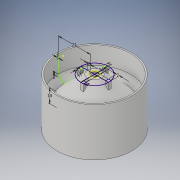
# Autodesk Inventor part: flyflipfunnel
Saved by Autodesk Inventor 2019 (Build 230136000, 136)
## iProperties
Created: 2019-02-13
Part Number: flyflipfunnel
Material: Generic
Document SubType Name: Modeling
Designer: rhaase
Density: 1 g/cm^3
Appearance: Default
Author: rhaase
Autodesk Inventor part; units mm, degrees
ref_plane "YZ Plane" through (0, 0, 0) normal (1, 0, 0) x (0, 1, 0)
ref_plane "XZ Plane" through (0, 0, 0) normal (0, 1, 0) x (-1, 0, 0)
ref_plane "XY Plane" through (0, 0, 0) normal (0, 0, 1) x (1, 0, 0)
sketch "Sketch1" plane through (0, 0, 0) normal (0, 0, 1) x (1, 0, 0)
  line L0 (-3.313, 2.109) -> (-3.313, 22.109)
  line L1 (-3.313, 4.109) -> (-3.313, 2.109)
  line L2 (22.687, -0.5116) -> (12.687, 9.4884)
  line L3 (12.687, 9.4884) -> (12.687, 7.4884)
  line L4 (12.687, 7.4884) -> (22.687, -2.5116)
  line L5 (22.687, -2.5116) -> (22.687, -0.5116)
  line L6 (-0.313, 2.109) -> (19.687, 22.109)
  line L7 (19.687, 22.109) -> (17.687, 22.109)
  line L8 (17.687, 22.109) -> (-0.313, 4.109)
  line L9 (12.187, 14.609) -> (13.6012, 16.0232)
  line L10 (-0.313, 2.109) -> (19.687, 22.109)
  line L11 (17.687, 22.109) -> (-0.313, 4.109)
  line L12 (-0.313, 4.109) -> (-0.313, 2.109)
  line L13 (19.687, 22.109) -> (17.687, 22.109)
  line L14 (-0.313, 4.109) -> (-0.313, 2.109)
  line L15 (-0.313, 2.109) -> (19.687, 22.109)
  line L16 (17.687, 22.109) -> (-0.313, 4.109)
  line L17 (-0.313, 4.109) -> (-3.313, 7.109)
  line L18 (-3.313, 22.109) -> (-4.313, 22.109)
  line L19 (-3.313, 7.109) -> (-3.313, 9.109)
  line L20 (-3.313, 9.109) -> (0.687, 5.109)
  line L21 (-3.313, 7.109) -> (-3.313, -2.5116)
  line L22 (-4.313, -2.5116) -> (-4.313, 22.109)
  line L23 (-3.313, 22.109) -> (-3.313, 9.109)
  line L24 (-4.313, -2.5116) -> (-3.313, -2.5116)
  line L25 (-4.313, -2.5116) -> (-4.313, -12.5116)
  line L26 (-4.313, -12.5116) -> (-3.313, -12.5116)
  line L27 (-3.313, -12.5116) -> (-3.313, -2.5116)
  line L28 (-0.313, 2.109) -> (-3.313, -0.891)
  line L29 (-3.313, 1.109) -> (-0.313, 4.109)
  dimension "d20" = 2
  dimension "d21" = 2
  dimension "d50" = 1
  dimension "d67" = 23
  dimension "d69" = 2
  dimension "d71" = 10
  constraints: 60 end point, 6 point on line, 4 parallel, 3 horizontal, 3 perpendicular, 2 collinear, 1 vertical
  measures "d20" distance of L6.end L7.end
  measures "d21" distance of L9.start L9.end
  measures "d50" distance of L0.end L18.end
  measures "d67" distance of L0.end L6.end
  measures "d69" distance of L17.end L19.end
  measures "d71" distance of L22.start L25.end
revolve "Revolution4" add sketch "Sketch1" angle 360 about axis through (22.687, -2.5116, 0) along (0, 1, 0) contours L8 L7 L6 L12
sketch "Sketch2" plane through (22.687, 22.109, 0) normal (0, 1, 0) x (1, 0, 0)
  circle A0 centre (0, 0) radius 3 projected
  circle A1 centre (0, 0) radius 10
  line L0 (0, 0) -> (10, 0)
  circle A2 centre (0, 0) radius 10 projected
  line L1 (0, 0) -> (0, -10)
  line L2 (0, 0) -> (0, -10)
  line L3 (0, 0) -> (-10, 0)
  line L4 (0, 0) -> (0, 10)
  line L5 (0, -8) -> (0, -10)
  line L6 (0, -8) -> (0, -10)
  line L7 (10, 0) -> (8, 0)
  line L8 (8, 0) -> (8, 2)
  line L9 (8, 2) -> (10, 2)
  line L10 (10, 2) -> (10, 0)
  line L11 (0, 8) -> (0, 10)
  line L12 (-10, 0) -> (-8, 0)
  line L13 (-8, 0) -> (-8, -2)
  line L14 (-8, -2) -> (-10, -2)
  line L15 (-10, -2) -> (-10, 0)
  line L16 (0, 8) -> (0, 10)
  line L17 (0, 8) -> (-2, 8)
  line L18 (-2, 8) -> (-2, 10)
  line L19 (-2, 10) -> (0, 10)
  line L20 (0, 10) -> (0, 8)
  line L21 (0, -10) -> (2, -10)
  line L22 (2, -10) -> (2, -8)
  line L23 (2, -8) -> (0, -8)
  line L24 (0, -8) -> (0, -10)
  point P0 (-22.687, 0)
  dimension "d29" = 20
  dimension "d34" = 2
  dimension "d35" = 2
  dimension "d54" = 2
  dimension "d56" = 2
  dimension "d57" = 2
  constraints: 50 end point, 8 parallel, 6 horizontal, 6 perpendicular, 3 point on circle, 1 coincident, 1 vertical, 1 vertical alignment, 2 other
  measures "d34" distance of L8.end L9.end
  measures "d35" distance of L7.end L8.end
  measures "d54" distance of L18.end L19.end
  measures "d56" distance of L23.end L22.end
  measures "d57" distance of L22.end L21.end
revolve "Revolution10" add sketch "Sketch1" angle 360 about axis through (22.687, -2.5116, 0) along (0, 1, 0) contours L5 L4 L3 L2
extrude "Extrusion5" add sketch "Sketch2" against normal blind 14 contours L17 L18 A1 L4 | A1 L18 L19
extrude "Extrusion6" add sketch "Sketch2" against normal blind 14 contours L23 L22 A1 L1 | A1 L22 L21
extrude "Extrusion7" add sketch "Sketch2" against normal blind 14 contours L13 L14 A1 L3 | A1 L14 L15
extrude "Extrusion8" add sketch "Sketch2" against normal blind 14 contours L8 L9 A1 L0 | A1 L9 L10
revolve "Revolution11" add sketch "Sketch1" angle 360 about axis through (22.687, -2.5116, 0) along (0, 1, 0) contours L21 L24 L22 L18 L0 | L0 L20 L8 L17
sketch "Sketch3" plane through (22.687, -2.5116, 0) normal (0, -1, 0) x (1, 0, 0)
  point P0 (-22.687, 0)
revolve "Revolution12" add sketch "Sketch1" angle 360 about axis through (22.687, -2.5116, 0) along (0, 1, 0) contours L21 L24 L22 L18 L0 | L29 L12 L28 L21 | L27 L26 L25 L24
body "Solid1"
